insert (Autodesk Fusion 360 design; units mm, degrees)
Autodesk Fusion 360 part; units mm, degrees
note: some values were not read from the file. Set by a fixed rule: which sketch regions a step uses.
sketch "Sketch1" plane through (0, 0, 0) normal (0, 1, 0) x (1, 0, 0)
  circle A0 centre (10.4669, -3.4) radius 2.5
  spline S0 degree 5 poles (11.9078, -1.357) (11.8765, -1.3273) (11.8232, -1.2692) (11.7712, -1.1858) (11.7579, -1.0822) (11.8332, -0.9664) (11.9946, -0.8671) (12.2294, -0.7894) (12.5196, -0.7412) (12.8437, -0.7327) (13.1786, -0.7763) (13.5005, -0.8867) (13.787, -1.0776) (14.0182, -1.3587) (14.1778, -1.7326) (14.2555, -2.1915) (14.2463, -2.7169) (14.1497, -3.2833) (13.968, -3.8612) (13.7058, -4.4201) (13.3687, -4.9309) (12.9619, -5.3695) (12.4902, -5.7191) (11.957, -5.9687) (11.3654, -6.1117) (10.7172, -6.1451) (10.1546, -6.0833) (9.7082, -5.9875) (9.3998, -5.9015) (9.2429, -5.8531) knots 0 0 0 0 0 0 0.04 0.08 0.12 0.16 0.2 0.24 0.28 0.32 0.36 0.4 0.44 0.48 0.52 0.56 0.6 0.64 0.68 0.72 0.76 0.8 0.84 0.88 0.92 0.96 1 1 1 1 1 1
  spline S1 degree 5 poles (11.3443, -1.059) (11.3773, -1.0732) (11.4422, -1.0961) (11.5368, -1.114) (11.6573, -1.1047) (11.7956, -1.0389) (11.9126, -0.9224) (11.9895, -0.7644) (11.9995, -0.5791) (11.9167, -0.3828) (11.7224, -0.1922) (11.4147, -0.0213) (11.006, 0.1187) (10.5186, 0.2187) (9.98, 0.2718) (9.4196, 0.273) (8.8649, 0.2188) (8.3366, 0.1074) (7.8483, -0.0616) (7.4085, -0.2878) (7.0213, -0.5702) (6.7551, -0.8405) (6.58, -1.0678) (6.4741, -1.2301) (6.4239, -1.314) knots 0 0 0 0 0 0 0.05 0.1 0.15 0.2 0.25 0.3 0.35 0.4 0.45 0.5 0.55 0.6 0.65 0.7 0.75 0.8 0.85 0.9 0.95 1 1 1 1 1 1
  spline S2 degree 5 poles (13.3936, -4.858) (13.4507, -4.7929) (13.5609, -4.6568) (13.7138, -4.4347) (13.893, -4.1029) (14.077, -3.6299) (14.2247, -3.104) (14.3444, -2.536) (14.4494, -1.944) (14.5611, -1.3563) (14.7041, -0.8082) (14.8994, -0.3359) (15.1576, 0.029) (15.4733, 0.2641) (15.8153, 0.3632) (16.13, 0.3373) (16.3642, 0.2064) (16.4833, -0.0062) (16.4938, -0.2812) (16.4289, -0.6036) (16.3301, -0.9625) (16.228, -1.3512) (16.1315, -1.7663) (16.0367, -2.206) (15.9307, -2.6677) (15.7971, -3.1468) (15.6216, -3.6344) (15.3937, -4.1172) (15.1051, -4.58) (14.7503, -5.0066) (14.3253, -5.3818) (13.8274, -5.6928) (13.2551, -5.9305) (12.6074, -6.0887) (11.8841, -6.1637) (11.0852, -6.1533) (10.3858, -6.0762) (9.8274, -5.9797) (9.4402, -5.8981) (9.2429, -5.8531) knots 0 0 0 0 0 0 0.028571 0.057143 0.085714 0.114286 0.142857 0.171429 0.2 0.228571 0.257143 0.285714 0.314286 0.342857 0.371429 0.4 0.428571 0.457143 0.485714 0.514286 0.542857 0.571429 0.6 0.628571 0.657143 0.685714 0.714286 0.742857 0.771429 0.8 0.828571 0.857143 0.885714 0.914286 0.942857 0.971429 1 1 1 1 1 1
  spline S3 degree 5 poles (9.2429, -5.8531) (9.4775, -5.9537) (9.9363, -6.1391) (10.5936, -6.3697) (11.4078, -6.582) (12.3229, -6.6884) (13.1407, -6.637) (13.8728, -6.4325) (14.5405, -6.0842) (15.1751, -5.6087) (15.8292, -5.0295) (16.4928, -4.4062) (17.1259, -3.8086) (17.6765, -3.2989) (18.1025, -2.9098) (18.3948, -2.6269) (18.5975, -2.3594) (18.6818, -2.0553) (18.6087, -1.7116) (18.3565, -1.43) (17.9457, -1.382) (17.4181, -1.7067) (16.835, -2.3298) (16.2504, -3.0407) (15.6965, -3.7493) (15.1932, -4.3836) (14.8384, -4.8095) (14.6005, -5.0778) (14.4543, -5.2342) (14.3844, -5.3068) knots 0 0 0 0 0 0 0.04 0.08 0.12 0.16 0.2 0.24 0.28 0.32 0.36 0.4 0.44 0.48 0.52 0.56 0.6 0.64 0.68 0.72 0.76 0.8 0.84 0.88 0.92 0.96 1 1 1 1 1 1
  line L0 (18.5608, -0.7824) -> (16.1848, -2.8314)
  line L1 (13.8339, -6.5816) -> (15.9045, -5.0647)
  spline S4 degree 5 poles (9.2429, -5.8531) (9.4448, -5.9589) (9.8467, -6.1578) (10.4434, -6.4181) (11.2266, -6.6886) (12.1862, -6.8981) (13.1297, -6.9782) (14.0662, -6.9301) (15.0078, -6.7588) (15.98, -6.4728) (17.0067, -6.0896) (17.9733, -5.6499) (18.7277, -5.2029) (19.1657, -4.785) (19.2344, -4.4321) (19.1833, -4.1021) (19.0173, -3.8851) (18.5109, -3.9502) (17.5896, -4.351) (16.4311, -4.9664) (15.3388, -5.5884) (14.7926, -5.9025) (14.6947, -5.9473) (14.7851, -5.8806) (14.8692, -5.8232) knots 0 0 0 0 0 0 0.05 0.1 0.15 0.2 0.25 0.3 0.35 0.4 0.45 0.5 0.55 0.6 0.65 0.7 0.75 0.8 0.85 0.9 0.95 1 1 1 1 1 1
  line L2 (14.5476, -6.043) -> (15.1907, -5.6034)
  line L3 (19.1172, -5.0553) -> (19.2758, -3.9419)
  line L4 (-6.0412, -6.8423) -> (-6.0412, -0.0423)
  line L5 (-6.0412, -6.8423) -> (-1.0412, -6.8423)
  line L6 (-1.0412, -6.8423) -> (-1.0412, -6.014)
  line L7 (-1.0412, -6.014) -> (6, -6.014)
  line L8 (-6.0412, -0.0423) -> (-1.0412, -0.0423)
  line L9 (-1.0412, -0.0423) -> (-1.0412, -1.314)
  line L10 (-1.0412, -1.314) -> (6.4239, -1.314)
  spline S5 degree 5 poles (6, -6.014) (6.0769, -6.068) (6.2341, -6.1741) (6.4802, -6.3275) (6.829, -6.5208) (7.3003, -6.7426) (7.8077, -6.9429) (8.3515, -7.1188) (8.9309, -7.2661) (9.5439, -7.3798) (10.1881, -7.4544) (10.8609, -7.4848) (11.5596, -7.4673) (12.2818, -7.4) (13.0254, -7.2833) (13.7889, -7.1183) (14.4146, -6.9488) (14.892, -6.8011) (15.2138, -6.6935) (15.3756, -6.6375) knots 0 0 0 0 0 0 0.066667 0.133333 0.2 0.266667 0.333333 0.4 0.466667 0.533333 0.6 0.666667 0.733333 0.8 0.866667 0.933333 1 1 1 1 1 1
  line L11 (14.1094, -6.9877) -> (16.6419, -6.2873)
  line L12 (17.5, -3.5) -> (18.9077, -2.113)
  point P0 (11.8529, -0.9721)
  point P1 (12.8153, -0.7442)
  point P2 (14.0843, -1.5472)
  point P3 (13.3936, -4.858)
  point P4 (11.8529, -0.9721)
  point P5 (11.8529, -0.339)
  point P6 (9.1937, 0.2435)
  point P7 (14.3754, -2.3508)
  point P8 (15.3572, 0.1564)
  point P9 (16.3571, 0.1637)
  point P10 (16.3644, -0.8363)
  point P11 (15.879, -2.8398)
  point P12 (14.3844, -5.3068)
  point P13 (14.8692, -5.8232)
  point P14 (18.2039, -2.8065)
  point P15 (18.6132, -1.8446)
  point P16 (17.3728, -1.8069)
  point P17 (15.3756, -6.6375)
  point P18 (19.1965, -4.4986)
  point P19 (18.6355, -3.9708)
  point P20 (8, -7)
  point P21 (11.0651, -7.4727)
  point P22 (16.0251, -4.8413)
  dimension "d3" = 5
  dimension "d7" = 6.8
  dimension "d9" = 4.7
  dimension "d10" = 5
  dimension "d11" = 5
  constraint coincident A0 S0.start
  constraint coincident A0 S1.start
  constraint coincident P4 P0
  constraint coincident P3 S2.start
  constraint coincident P12 S3.end
  constraint midpoint P16 L0
  constraint midpoint P13 L1
  constraint coincident P13 S4.end
  constraint midpoint P13 L2
  constraint coincident S3 L2.start
  constraint midpoint P18 L3
  constraint vertical L4
  constraint perpendicular L4 L5
  constraint perpendicular L5 L6
  constraint perpendicular L6 L7
  constraint perpendicular L4 L8
  constraint perpendicular L8 L9
  constraint perpendicular L9 L10
  constraint coincident S1.end L10.end
  constraint coincident P17 S5.end
  constraint midpoint P17 L11
  constraint midpoint P14 L12
  measures "d3" diameter of A0
  measures "d7" distance of L4.start L4.end
  measures "d9" vertical distance of L6.end L9.end
  measures "d10" distance of L4.start L5.end
  measures "d11" distance of L4.end L8.end
extrude "Extrude2" add sketch "Sketch1" along normal blind 1.35 makes body 1
sketch "Sketch2" plane through (0, 0, 0) normal (0, 1, 0) x (1, 0, 0)
  circle A0 centre (13.2, -6.1) radius 0.75
  dimension "d16" = 1.5
  measures "d16" diameter of A0
extrude "Extrude3" add sketch "Sketch2" against normal blind 0.65 separate body makes body 2
